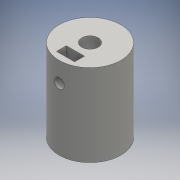
# Autodesk Inventor part: MotorTripodCoupler
Saved by Autodesk Inventor 2016 (Build 200138000, 138)
## iProperties
Created: 2016-05-22
Part Number: MotorTripodCoupler
Material: Generic
Document SubType Name: Modeling
Designer: Kurtis
Density: 1 g/cm^3
Appearance: Default
Author: Kurtis
Autodesk Inventor part; units mm, degrees
ref_plane "YZ Plane" through (0, 0, 0) normal (1, 0, 0) x (0, 1, 0)
ref_plane "XZ Plane" through (0, 0, 0) normal (0, 1, 0) x (-1, 0, 0)
sketch "Sketch1" plane through (0, 0, 0) normal (0, 0, 1) x (1, 0, 0)
  circle A0 centre (0, 0) radius 9.375
  circle A1 centre (0, 0) radius 2.5
  dimension "d0" = 18.75
  dimension "d1" = 5
  constraints: 2 centre point, 2 coincident
  measures "d0" diameter of A0
  measures "d1" diameter of A1
extrude "Extrusion1" add sketch "Sketch1" along normal blind 25
sketch "Point of Tangency + Nut" plane through (0, 0, 25) normal (0, 0, 1) x (1, 0, 0)
  circle A0 centre (0, 0) radius 9.375 projected
  line L0 (0, -9.375) -> (0, -2.5) construction
  circle A1 centre (0, 0) radius 2.5 construction
  line L1 (2.75, -7.4375) -> (-2.75, -7.4375)
  line L2 (-2.75, -7.4375) -> (-2.75, -4.4375)
  line L3 (-2.75, -4.4375) -> (2.75, -4.4375)
  line L4 (2.75, -4.4375) -> (2.75, -7.4375)
  line L5 (2.75, -7.4375) -> (-2.75, -4.4375) construction
  line L6 (-2.75, -7.4375) -> (2.75, -4.4375) construction
  point P0 (0, -5.9375)
  dimension "d8" = 5.5
  dimension "d9" = 3
  constraints: 14 end point, 3 midpoint, 2 parallel, 2 vertical alignment, 1 horizontal, 1 perpendicular, 1 vertical, 2 other
  measures "d8" distance of L2.end L3.end
  measures "d9" distance of L1.end L2.end
ref_plane "Work Plane1" through (0, -9.375, 25) normal (0, -1, 0) x (1, 0, 0)
sketch "Sketch3" plane through (0, -9.375, 25) normal (0, -1, 0) x (1, 0, 0)
  line L0 (9.375, 0) -> (-9.375, 0) construction
  line L1 (0, 0) -> (0, -6) construction
  circle A0 centre (0, -6) radius 1.5
  point P0 (0, -25)
  dimension "d4" = 6
  dimension "d5" = 3
  constraints: 2 end point, 1 centre point, 1 coincident, 1 midpoint, 1 vertical
  measures "d4" distance of L1.start L1.end
  measures "d5" diameter of A0
extrude "LocBolt" cut sketch "Sketch3" against normal blind 8
extrude "LocNut Gap" cut sketch "Point of Tangency + Nut" against normal blind 9.5 contours L1 L2 L3 L4
body "Solid1"
